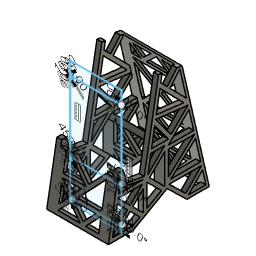
OpenStand V1 (Autodesk Fusion 360 design; units mm, degrees)
Autodesk Fusion 360 part; units mm, degrees
sketch "Sketch1" plane through (0, 0, 0) normal (1, 0, 0) x (0, 1, 0)
  line L0 (0, 0) -> (2.7266, 0)
  line L1 (2.7266, 0) -> (71.6615, -12.165)
  line L2 (71.6615, -12.165) -> (132.4864, 332.5093)
  line L3 (132.4864, 332.5093) -> (221.1169, 316.8686)
  line L4 (221.1169, 316.8686) -> (335.0057, -179.6839)
  line L5 (335.0057, -179.6839) -> (244.5254, -179.6839)
  line L6 (244.5254, -179.6839) -> (164.179, -101.509)
  line L7 (-73.965, -179.6839) -> (-33.062, 52.0995)
  line L8 (-33.062, 52.0995) -> (-13.7716, 52.8108)
  line L9 (-13.7716, 52.8108) -> (0, 0)
  line L10 (-73.965, -179.6839) -> (26.035, -179.6839)
  line L11 (26.035, -179.6839) -> (164.179, -101.509)
  line L12 (-57.1941, -163.3688) -> (-23.4168, 28.0357)
  line L13 (-23.4168, 28.0357) -> (-14.2489, -7.1211)
  line L14 (-14.2489, -7.1211) -> (84.2295, -24.4996)
  line L15 (84.2295, -24.4996) -> (143.8137, 313.1445)
  line L16 (143.8137, 313.1445) -> (214.1563, 300.7311)
  line L17 (214.1563, 300.7311) -> (321.4409, -167.0272)
  line L18 (321.4409, -167.0272) -> (250.587, -167.0272)
  line L19 (250.587, -167.0272) -> (164.9021, -83.6581)
  line L20 (164.9021, -83.6581) -> (24.0441, -163.3688)
  line L21 (24.0441, -163.3688) -> (-57.1941, -163.3688)
  line L22 (-57.1941, -163.3688) -> (139.7385, -163.3688) construction
  line L23 (-57.1941, -163.3688) -> (-42.1941, -163.3688)
  line L24 (-42.1941, -163.3688) -> (252.9158, 131.741)
  line L25 (-42.1941, -163.3688) -> (375.1543, -163.3688) construction
  line L26 (-42.1941, -163.3688) -> (14.3745, -106.8003)
  line L27 (14.3745, -106.8003) -> (53.9943, -146.4202)
  line L28 (14.3745, -106.8003) -> (24.9811, -96.1937)
  line L29 (24.9811, -96.1937) -> (67.5413, -138.754)
  line L30 (-42.1941, -163.3688) -> (-52.8007, -152.7622)
  line L31 (-52.8007, -152.7622) -> (248.9581, 148.9965)
  line L32 (-52.8007, -152.7622) -> (-55.3223, -152.7622)
  line L33 (3.7679, -96.1937) -> (14.3745, -85.5871)
  line L34 (14.3745, -85.5871) -> (-34.7915, -36.4211)
  line L35 (3.7679, -96.1937) -> (-37.9735, -54.4523)
  line L36 (-34.7915, -36.4211) -> (63.5405, -36.4211)
  line L37 (63.5405, -21.4211) -> (66.7846, -21.4211)
  line L38 (63.5405, -21.4211) -> (-32.1445, -21.4211)
  line L39 (67.5413, -138.754) -> (67.5413, -53.6334)
  line L40 (82.5413, -130.2656) -> (82.5413, -38.6334)
  line L41 (82.5413, -38.6334) -> (141.0588, -97.1509)
  line L42 (82.5413, -38.6334) -> (93.1479, -28.0268)
  line L43 (93.1479, -28.0268) -> (154.6058, -89.4847)
  line L44 (154.6058, -89.4847) -> (154.6058, 33.431)
  line L45 (169.6014, -88.2303) -> (169.6014, 48.4266)
  line L46 (154.6058, 54.6442) -> (98.196, 54.6442)
  line L47 (169.6014, 69.6398) -> (100.8423, 69.6398)
  line L48 (250.587, -167.0272) -> (307.9247, -108.0968)
  line L49 (250.587, -167.0272) -> (239.8361, -156.5669)
  line L50 (239.8361, -156.5669) -> (303.9324, -90.6902)
  line L51 (303.9324, -90.6902) -> (172.1296, -90.6902)
  line L52 (169.6014, -75.6902) -> (300.492, -75.6902)
  line L53 (179.1877, -75.6902) -> (279.2876, 16.7605)
  line L54 (169.6014, -64.1532) -> (275.4283, 33.5869)
  line L55 (275.4283, 33.5869) -> (169.6014, 33.5869)
  line L56 (169.6014, 33.5869) -> (169.6014, 48.5869)
  line L57 (169.6014, 48.5869) -> (271.9879, 48.5869)
  line L58 (169.6014, 69.6398) -> (114.0216, 144.3225)
  line L59 (180.3214, 80.3598) -> (117.6055, 164.6314)
  line L60 (117.6055, 164.6314) -> (248.9581, 148.9965)
  line L61 (245.3961, 164.5263) -> (120.2164, 179.4265)
  line L62 (242.617, 176.6434) -> (138.4371, 282.6772)
  line L63 (231.9173, 166.1307) -> (135.2353, 264.5333)
  line L64 (204.5607, 302.4245) -> (164.9125, 255.7307)
  line L65 (215.9948, 292.7157) -> (175.4681, 244.9873)
  line L66 (-23.4168, 28.0357) -> (-36.889, 30.4131)
  arc A0 (-57.1941, -163.3688) -> (-57.1941, -166.1272) centre (-49.3789, -164.748) ccw
  line L67 (-57.1941, -166.1272) -> (-57.1941, -179.6839)
  line L68 (143.8137, 313.1445) -> (129.5144, 315.668)
  line L69 (214.1563, 300.7311) -> (225.2679, 298.7703)
  line L70 (321.4409, -167.0272) -> (324.3439, -179.6839)
  dimension "d1" = 70
  dimension "d2" = 350
  dimension "d3" = 90
  dimension "d4" = 100
  dimension "d6" = 100
  dimension "d8" = 15
  dimension "d9" = 45
  dimension "d10" = 80
  dimension "d11" = 15
  dimension "d12" = 15
  dimension "d13" = 15
  dimension "d14" = 15
  dimension "d16" = 15
  dimension "d18" = 15
  dimension "d20" = 15
  dimension "d21" = 15
  dimension "d24" = 15
  dimension "d25" = 15
  constraint coincident L0.start L9.end
  constraint horizontal L0
  constraint perpendicular L1 L2
  constraint perpendicular L2 L3
  constraint horizontal L5
  constraint parallel L2 L7
  constraint horizontal L10
  constraint parallel L7 L12
  constraint parallel L9 L13
  constraint perpendicular L2 L14
  constraint perpendicular L14 L15
  constraint perpendicular L15 L16
  constraint parallel L4 L17
  constraint horizontal L18
  constraint parallel L6 L19
  constraint parallel L11 L20
  constraint horizontal L21
  constraint horizontal L22
  constraint coincident L22 L23.end
  constraint horizontal L25
  constraint coincident L17 L24.end
  constraint parallel L24 L26
  constraint coincident L20 L27.end
  constraint perpendicular L26 L27
  constraint perpendicular L27 L28
  constraint coincident L20 L29.end
  constraint perpendicular L24 L29
  constraint coincident L17 L31.end
  constraint perpendicular L30 L31
  constraint coincident L12 L32.end
  constraint horizontal L32
  constraint coincident L31 L33.start
  constraint parallel L31 L33
  constraint coincident L12 L34.end
  constraint perpendicular L31 L34
  constraint coincident L12 L35.end
  constraint perpendicular L33 L35
  constraint coincident L31 L36.end
  constraint horizontal L36
  constraint coincident L14 L37.end
  constraint coincident L12 L38.end
  constraint coincident L24 L39.end
  constraint vertical L39
  constraint coincident L24 L40.end
  constraint coincident L20 L40.start
  constraint coincident L20 L41.end
  constraint perpendicular L24 L41
  constraint perpendicular L41 L42
  constraint coincident L20 L43.end
  constraint perpendicular L24 L43
  constraint coincident L24 L44.end
  constraint vertical L44
  constraint coincident L24 L45.end
  constraint coincident L19 L45.start
  constraint coincident L31 L46.start
  constraint coincident L15 L46.end
  constraint perpendicular L44 L46
  constraint coincident L31 L47.start
  constraint coincident L15 L47.end
  constraint parallel L46 L47
  constraint coincident L17 L48.end
  constraint perpendicular L19 L48
  constraint perpendicular L48 L49
  constraint coincident L17 L50.end
  constraint perpendicular L19 L50
  constraint coincident L19 L51.end
  constraint horizontal L51
  constraint coincident L45 L52.start
  constraint coincident L17 L52.end
  constraint coincident L45 L54.start
  constraint coincident L52 L53.start
  constraint coincident L17 L53.end
  constraint coincident L17 L54.end
  constraint parallel L53 L54
  constraint coincident L45 L55.end
  constraint perpendicular L45 L55
  constraint perpendicular L55 L56
  constraint coincident L17 L57.end
  constraint perpendicular L45 L57
  constraint midpoint L15 L58.end
  constraint coincident L15 L59.end
  constraint coincident L31 L59.start
  constraint coincident L17 L61.start
  constraint coincident L15 L61.end
  constraint coincident L61 L63.start
  constraint coincident L17 L62.start
  constraint coincident L15 L62.end
  constraint coincident L15 L63.end
  constraint coincident L17 L65.start
  constraint coincident L16 L64.start
  constraint coincident L62 L64.end
  constraint coincident L62 L65.end
  constraint coincident L7 L66.end
  constraint perpendicular L7 L66
  constraint tangent L12 A0
  constraint coincident L10 L67.end
  constraint perpendicular L10 L67
  constraint coincident L2 L68.end
  constraint perpendicular L2 L68
  constraint coincident L4 L69.end
  constraint parallel L16 L69
  constraint parallel L17 L70
  measures "d1" distance of L0.end L1.end
  measures "d2" distance of L1.end L2.end
  measures "d3" distance of L2.end L3.end
  measures "d4" distance of L7.start L10.end
  measures "d6" distance of L13.end L14.end
  measures "d8" distance of L12.start L23.end
  measures "d9" angle of L24 L25
  measures "d10" distance of L23.end L26.end
  measures "d11" distance of L26.end L28.end
  measures "d12" distance of L23.end L30.end
  measures "d13" distance of L33.start L33.end
  measures "d14" distance of L36.end L37.start
  measures "d16" distance of L40.end L42.end
  measures "d18" distance of L18.end L49.end
  measures "d20" distance of L54.start L53.start
  measures "d21" distance of L55.end L56.end
  measures "d24" distance of L63.start L62.start
  measures "d25" distance of L65.start L64.start
extrude "Extrude1" add sketch "Sketch1" along normal blind 20 contours L0 L1 L2 L7 L8 L9 L13 L14 L15 L31 L66 L68 | L15 L17 L61 L62 L63 | L16 L17 L62 L64 L65 | L5 L6 L10 L11 L18 L19 L20 L21 L23 L49 A0 L67 L70 | L12 L14 L31 L36 L37 L38 | L12 L31 L33 L34 L35 | L15 L17 L60 L61 | L12 L21 L23 L30 L32 | L14 L15 L17 L24 L26 L28 L30 L31 L33 L42 L56 L57 | L14 L15 L31 | L15 L31 L58 L59 | L20 L24 L27 L28 L29 | L15 L31 L46 L47 | L17 L19 L48 L49 L50 | L17 L19 L45 L51 L52 | L17 L24 L45 L55 L56 L57 | L20 L24 L39 L40 | L17 L45 L52 L53 L54 | L20 L24 L41 L42 L43
extrude "Extrude2" add sketch "Sketch1" along normal blind 250 contours L7 L10 L12 L66 A0 L67 | L4 L5 L17 L69 L70 | L19 L20 L24 L44 L45 L56
extrude "Extrude3" add sketch "Sketch1" along normal blind 250 and the other way blind -230 contours L0 L1 L2 L7 L8 L9 L13 L14 L15 L31 L66 L68 | L15 L17 L61 L62 L63 | L16 L17 L62 L64 L65 | L5 L6 L10 L11 L18 L19 L20 L21 L23 L49 A0 L67 L70 | L12 L14 L31 L36 L37 L38 | L12 L31 L33 L34 L35 | L15 L17 L60 L61 | L14 L15 L17 L24 L26 L28 L30 L31 L33 L42 L56 L57 | L14 L15 L31 | L15 L31 L58 L59 | L20 L24 L27 L28 L29 | L15 L31 L46 L47 | L17 L19 L48 L49 L50 | L17 L19 L45 L51 L52 | L17 L24 L45 L55 L56 L57 | L20 L24 L39 L40 | L17 L45 L52 L53 L54 | L20 L24 L41 L42 L43
sketch "Sketch2" plane through (0, 0, 0) normal (0, 1, 0) x (1, 0, 0)
  line L0 (27.6259, 180.2965) -> (225.1194, -29.8221)
  line L1 (225.1194, -29.8221) -> (204.5336, -29.8221)
  line L2 (27.6259, 180.2965) -> (225.1194, 180.2965)
  line L3 (225.1194, 180.2965) -> (225.1194, -29.8221)
  line L4 (22.161, -29.8221) -> (22.161, 164.2091)
  line L5 (22.161, 164.2091) -> (27.6259, 180.2965)
  line L6 (22.161, 164.2091) -> (204.5336, -29.8221)
  line L7 (22.161, 164.2091) -> (22.161, 180.2965)
  line L8 (22.161, 180.2965) -> (27.6259, 180.2965)
  line L9 (42.7467, 164.2091) -> (207.8462, 164.2091)
  line L10 (207.8462, 164.2091) -> (207.8462, -11.4447)
  line L11 (42.7467, -12.4948) -> (42.7467, 164.2091)
  line L12 (132.3063, 164.2091) -> (42.7467, 80.0308)
  line L13 (132.3063, 164.2091) -> (142.5794, 153.2792)
  line L14 (142.5794, 153.2792) -> (154.208, 164.2091)
  line L15 (142.5794, 153.2792) -> (42.7467, 59.445)
  line L16 (42.7467, -12.4948) -> (42.7467, -301.0302)
  line L17 (22.161, -29.8221) -> (22.161, -301.0302)
  line L18 (22.161, -301.0302) -> (42.7467, -301.0302)
  line L19 (225.1194, -29.8221) -> (225.1194, -301.0302)
  line L20 (225.1194, -301.0302) -> (207.8462, -301.0302)
  line L21 (207.8462, -301.0302) -> (207.8462, -11.4447)
  line L22 (204.5336, -29.8221) -> (207.8462, -33.3465)
  line L23 (154.208, 164.2091) -> (207.8462, 107.1419)
  line L24 (154.208, 164.2091) -> (143.2781, 153.9359)
  line L25 (143.2781, 153.9359) -> (207.8462, 85.2402)
  line L26 (95.0283, 108.5853) -> (185.9038, 108.5853)
  line L27 (185.9038, 108.5853) -> (185.9038, 93.5853)
  line L28 (185.9038, 93.5853) -> (109.1271, 93.5853)
  line L29 (185.9038, 93.5853) -> (200.0026, 93.5853)
  line L30 (42.7467, 59.445) -> (42.7467, 44.445)
  line L31 (42.7467, 44.445) -> (134.7289, 44.445)
  line L32 (42.7467, 59.445) -> (120.6302, 59.445)
  line L33 (134.7289, 44.445) -> (145.002, 33.5152)
  line L34 (145.002, 33.5152) -> (42.7467, -62.596)
  line L35 (134.7289, 44.445) -> (42.7467, -42.0103)
  line L36 (207.8462, -33.3465) -> (207.8462, -48.3465)
  line L37 (207.8462, -48.3465) -> (57.9072, -48.3465)
  line L38 (207.8462, -33.3465) -> (73.8661, -33.3465)
  line L39 (42.7467, -301.0302) -> (50.7595, -301.0302)
  line L40 (50.7595, -301.0302) -> (207.8462, -301.0302)
  line L41 (42.7467, -301.0302) -> (42.7467, -286.0302)
  line L42 (42.7467, -286.0302) -> (207.8462, -286.0302)
  line L43 (57.9072, -48.3465) -> (46.9773, -58.6196)
  line L44 (46.9773, -58.6196) -> (207.8462, -229.7724)
  line L45 (57.9072, -48.3465) -> (207.8462, -207.8707)
  line L46 (127.4118, -122.2943) -> (137.6849, -133.2242)
  line L47 (137.6849, -133.2242) -> (207.8462, -67.2786)
  line L48 (127.4118, -122.2943) -> (206.0868, -48.3465)
  line L49 (116.4819, -132.5674) -> (42.7467, -201.8722)
  line L50 (127.4118, -144.196) -> (42.7467, -223.7739)
  line L51 (42.7467, -223.7739) -> (42.7467, -238.7739)
  line L52 (42.7467, -238.7739) -> (207.8462, -238.7739)
  line L53 (42.7467, -223.7739) -> (202.2082, -223.7739)
  line L54 (207.8462, -248.9645) -> (173.5292, -286.0302)
  line L55 (196.8394, -238.7739) -> (153.0875, -286.0302)
  line L56 (153.0875, -286.0302) -> (102.0461, -238.7739)
  line L57 (131.0084, -286.0302) -> (79.967, -238.7739)
  line L58 (79.967, -238.7739) -> (90.9738, -248.9645)
  line L59 (90.9738, -248.9645) -> (56.6568, -286.0302)
  line L60 (79.967, -238.7739) -> (42.7467, -278.9754)
  dimension "d36" = 15
  dimension "d37" = 15
  dimension "d38" = 15
  dimension "d39" = 15
  dimension "d40" = 15
  dimension "d41" = 15
  dimension "d42" = 15
  dimension "d43" = 15
  dimension "d44" = 15
  dimension "d45" = 15
  dimension "d46" = 15
  dimension "d48" = 15
  constraint horizontal L1
  constraint parallel L1 L2
  constraint perpendicular L1 L3
  constraint parallel L0 L6
  constraint perpendicular L2 L7
  constraint perpendicular L7 L8
  constraint coincident L0 L9.start
  constraint perpendicular L3 L9
  constraint coincident L0 L10.end
  constraint perpendicular L9 L10
  constraint perpendicular L9 L11
  constraint coincident L9 L12.start
  constraint coincident L11 L12.end
  constraint perpendicular L6 L12
  constraint perpendicular L12 L13
  constraint coincident L9 L14.end
  constraint perpendicular L13 L14
  constraint coincident L11 L15.end
  constraint perpendicular L13 L15
  constraint vertical L16
  constraint parallel L16 L17
  constraint perpendicular L16 L18
  constraint perpendicular L18 L19
  constraint perpendicular L10 L20
  constraint perpendicular L20 L21
  constraint coincident L21 L22.end
  constraint parallel L6 L22
  constraint coincident L10 L23.end
  constraint perpendicular L14 L23
  constraint perpendicular L23 L24
  constraint coincident L10 L25.end
  constraint perpendicular L24 L25
  constraint coincident L15 L26.start
  constraint coincident L0 L26.start
  constraint coincident L25 L26.end
  constraint horizontal L26
  constraint perpendicular L26 L27
  constraint coincident L0 L28.end
  constraint perpendicular L27 L28
  constraint coincident L25 L29.end
  constraint perpendicular L27 L29
  constraint perpendicular L29 L30
  constraint coincident L6 L31.end
  constraint perpendicular L30 L31
  constraint coincident L6 L32.end
  constraint perpendicular L11 L32
  constraint parallel L6 L33
  constraint coincident L16 L34.end
  constraint perpendicular L33 L34
  constraint perpendicular L6 L35
  constraint parallel L21 L36
  constraint coincident L34 L37.end
  constraint perpendicular L36 L37
  constraint coincident L34 L38.end
  constraint perpendicular L21 L38
  constraint perpendicular L21 L40
  constraint perpendicular L20 L41
  constraint coincident L21 L42.end
  constraint perpendicular L21 L42
  constraint parallel L34 L43
  constraint coincident L21 L44.end
  constraint perpendicular L34 L44
  constraint coincident L21 L45.end
  constraint perpendicular L34 L45
  constraint coincident L45 L46.start
  constraint parallel L45 L46
  constraint coincident L21 L47.end
  constraint perpendicular L46 L47
  constraint coincident L37 L48.end
  constraint perpendicular L45 L48
  constraint coincident L44 L49.start
  constraint coincident L16 L49.end
  constraint perpendicular L44 L49
  constraint midpoint L44 L50.start
  constraint coincident L16 L50.end
  constraint perpendicular L44 L50
  constraint parallel L16 L51
  constraint coincident L21 L52.end
  constraint perpendicular L21 L52
  constraint coincident L44 L53.end
  constraint perpendicular L21 L53
  constraint coincident L52 L55.start
  constraint coincident L21 L54.start
  constraint coincident L42 L54.end
  constraint coincident L42 L55.end
  constraint coincident L52 L57.end
  constraint perpendicular L55 L56
  constraint coincident L42 L57.start
  constraint coincident L57 L58.end
  constraint coincident L42 L59.end
  constraint perpendicular L58 L59
  constraint coincident L16 L60.end
  constraint perpendicular L57 L60
  measures "d36" distance of L12.start L13.end
  measures "d37" distance of L14.end L24.end
  measures "d38" distance of L26.end L27.end
  measures "d39" distance of L15.end L30.end
  measures "d40" distance of L31.end L33.end
  measures "d41" distance of L22.end L36.end
  measures "d42" distance of L16.end L41.end
  measures "d43" distance of L37.end L43.end
  measures "d44" distance of L46.start L46.end
  measures "d45" distance of L50.end L51.end
  measures "d46" distance of L55.start L54.start
  measures "d48" distance of L57.end L58.end
extrude "Extrude4" cut sketch "Sketch2" along normal blind 410 and the other way blind 210 contours L0 L9 L12 | L6 L11 L12 | L14 L15 L25 L26 | L9 L10 L23 | L0 L10 L25 L28 L29 | L6 L15 L32 | L6 L22 L34 L38 | L11 L16 L31 L35 | L21 L42 L54 | L21 L45 L47 | L37 L45 L48 | L16 L52 L60 | L42 L57 L59 | L16 L34 L44 L49 | L52 L55 L56 | L44 L50 L53
sketch "Sketch3" plane through (0, 0, 0) normal (0, 1, 0) x (1, 0, 0)
  line L0 (20.5533, -315.7361) -> (20.5533, 181.7951)
  line L1 (229.3098, -315.7683) -> (229.3098, 184.781)
  line L2 (229.3098, 184.781) -> (20.5533, 181.7951)
  line L3 (20.5533, -315.7361) -> (229.3098, -315.7683)
  line L4 (229.3098, 184.781) -> (229.1098, 184.781)
  line L5 (229.1098, 184.781) -> (229.1098, -315.7682)
  line L6 (20.5533, 181.7951) -> (20.7533, 181.7951)
  line L7 (20.7533, 181.7951) -> (20.5533, -315.7361)
  line L8 (20.7477, 167.7878) -> (27.8188, 174.8589)
  line L9 (20.7477, 167.7878) -> (30.7477, 167.7878) construction
  line L10 (27.8188, 174.8589) -> (27.8188, 154.8589)
  line L11 (27.8188, 154.8589) -> (20.7454, 161.9276)
  line L12 (20.7454, 161.9276) -> (20.5533, 161.9276)
  line L13 (20.7477, 167.7878) -> (20.5533, 167.7878)
  line L14 (20.6878, 18.7874) -> (27.7589, 11.7163)
  line L15 (27.7589, 11.7163) -> (27.7669, 31.7163)
  line L16 (27.7669, 31.7163) -> (20.6902, 24.6509)
  line L17 (27.7629, 21.7163) -> (229.1098, 21.7163)
  line L18 (229.1098, 21.7163) -> (222.0358, 21.7163)
  line L19 (222.0358, 21.7163) -> (222.0358, 11.7163)
  line L20 (222.0358, 11.7163) -> (222.0358, 31.7163)
  line L21 (222.0358, 31.7163) -> (229.1098, 24.6423)
  line L22 (222.0358, 11.7163) -> (229.1098, 18.7903)
  line L23 (222.0358, 11.7163) -> (232.0399, 11.7163) construction
  line L24 (27.8188, 164.8589) -> (229.1098, 164.8589)
  line L25 (229.1098, 164.8589) -> (222.0358, 164.8589)
  line L26 (222.0358, 164.8589) -> (222.0358, 154.8589)
  line L27 (222.0358, 154.8589) -> (222.0358, 174.8589)
  line L28 (222.0358, 174.8589) -> (229.1098, 167.7849)
  line L29 (222.0358, 154.8589) -> (229.1098, 161.9329)
  line L30 (222.0358, 154.8589) -> (232.0399, 154.8589) construction
  line L31 (27.7629, -263.2837) -> (229.1098, -263.2837)
  line L32 (27.7589, -273.2837) -> (27.7669, -253.2837)
  line L33 (27.7669, -253.2837) -> (20.6902, -260.3491)
  line L34 (20.6878, -266.2126) -> (27.7589, -273.2837)
  line L35 (222.0358, -253.2837) -> (229.1098, -260.3577)
  line L36 (222.0358, -273.2837) -> (222.0358, -253.2837)
  line L37 (222.0358, -273.2837) -> (229.1098, -266.2097)
  line L38 (229.1098, -260.3577) -> (229.3098, -260.3577)
  line L39 (229.1098, -266.2097) -> (229.3098, -266.2097)
  line L40 (20.6902, -260.3491) -> (20.5533, -260.3491)
  line L41 (20.6878, -266.2126) -> (20.5533, -266.2126)
  line L42 (20.6902, 24.6509) -> (20.5533, 24.6509)
  line L43 (20.6878, 18.7874) -> (20.5533, 18.7874)
  line L44 (229.1098, 24.6423) -> (229.3098, 24.6423)
  line L45 (229.1098, 18.7903) -> (229.3098, 18.7903)
  line L46 (229.1098, 167.7849) -> (229.3098, 167.7849)
  line L47 (229.1098, 161.9329) -> (229.3098, 161.9329)
  dimension "d53" = 0.2
  dimension "d54" = 0.2
  dimension "d55" = 45
  dimension "d56" = 10
  dimension "d57" = 20
  dimension "d60" = 10
  dimension "d61" = 45
  dimension "d62" = 10
  dimension "d63" = 20
  dimension "d64" = 10
  dimension "d65" = 7.074
  dimension "d66" = 10
  dimension "d67" = 20
  dimension "d68" = 45
  dimension "d69" = 45
  dimension "d70" = 7.074
  dimension "d71" = 10
  dimension "d72" = 20
  dimension "d73" = 45
  dimension "d74" = 45
  dimension "d75" = 10
  dimension "d76" = 20
  dimension "d77" = 10
  dimension "d78" = 20
  dimension "d79" = 45
  constraint vertical L0
  constraint vertical L1
  constraint perpendicular L1 L4
  constraint vertical L5
  constraint coincident L3 L5.end
  constraint perpendicular L0 L6
  constraint horizontal L9
  constraint coincident L7 L8.start
  constraint perpendicular L9 L10
  constraint coincident L7 L11.end
  constraint coincident L0 L12.end
  constraint perpendicular L0 L12
  constraint coincident L0 L13.end
  constraint perpendicular L0 L13
  constraint coincident L7 L14.start
  constraint parallel L7 L15
  constraint coincident L7 L16.end
  constraint midpoint L15 L17.start
  constraint coincident L5 L17.end
  constraint perpendicular L5 L17
  constraint perpendicular L5 L18
  constraint perpendicular L17 L19
  constraint perpendicular L18 L20
  constraint coincident L5 L21.end
  constraint horizontal L23
  constraint coincident L5 L22.end
  constraint midpoint L10 L24.start
  constraint coincident L5 L24.end
  constraint perpendicular L5 L24
  constraint perpendicular L5 L25
  constraint perpendicular L24 L26
  constraint perpendicular L24 L27
  constraint coincident L5 L28.end
  constraint horizontal L30
  constraint coincident L5 L29.end
  constraint midpoint L31.start L32
  constraint coincident L1 L38.end
  constraint perpendicular L1 L38
  constraint coincident L1 L39.end
  constraint perpendicular L1 L39
  constraint coincident L0 L40.end
  constraint perpendicular L0 L40
  constraint coincident L0 L41.end
  constraint perpendicular L0 L41
  constraint coincident L0 L42.end
  constraint perpendicular L0 L42
  constraint coincident L0 L43.end
  constraint perpendicular L0 L43
  constraint coincident L1 L44.end
  constraint perpendicular L1 L44
  constraint coincident L1 L45.end
  constraint perpendicular L1 L45
  constraint coincident L1 L46.end
  constraint perpendicular L1 L46
  constraint coincident L1 L47.end
  constraint perpendicular L1 L47
  measures "d53" distance of L1.end L4.end
  measures "d54" distance of L0.end L6.end
  measures "d55" angle of L8 L9
  measures "d56" distance of L8.start L8.end
  measures "d57" distance of L8.end L10.end
  measures "d60" distance of L10.end L11.end
  measures "d61" angle of L13 L14
  measures "d62" distance of L14.start L14.end
  measures "d63" distance of L14.end L15.end
  measures "d64" distance of L15.end L16.end
  measures "d65" distance of L17.end L18.end
  measures "d66" distance of L18.end L19.end
  measures "d67" distance of L19.end L20.end
  measures "d68" angle of L20 L21
  measures "d69" angle of L22 L23
  measures "d70" distance of L24.end L25.end
  measures "d71" distance of L25.end L26.end
  measures "d72" distance of L26.end L27.end
  measures "d73" angle of L27 L28
  measures "d74" angle of L29 L30
  measures "d75" distance of L34.start L32.start
  measures "d76" distance of L32.start L32.end
  measures "d77" distance of L32.end L33.end
  measures "d78" distance of L36.start L35.start
  measures "d79" angle of L35 L36
